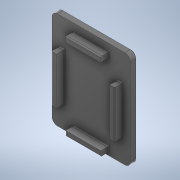
# Autodesk Inventor part: SP19V1 Tapacanto Delantero
Saved by Autodesk Inventor 2021.2 (Build 252289000, 289)
## iProperties
Created: 2026-06-08
Part Number: SP19V1 Tapacanto Delantero
Material: ABS Plastic
Document SubType Name: Modeling
Designer: NELSON
Density: 1.06 g/cm^3
Appearance: Smooth - Black
Author: NELSON
Autodesk Inventor part; units mm, degrees
ref_plane "YZ Plane" through (0, 0, 0) normal (1, 0, 0) x (0, 1, 0)
ref_plane "XZ Plane" through (0, 0, 0) normal (0, 1, 0) x (-1, 0, 0)
ref_plane "XY Plane" through (0, 0, 0) normal (0, 0, 1) x (1, 0, 0)
sketch "Boceto1" plane through (0, 0, 0) normal (0, 0, 1) x (1, 0, 0)
  line L0 (30, -40) -> (-30, -40)
  line L1 (-30, -40) -> (-30, 40)
  line L2 (-30, 40) -> (30, 40)
  line L3 (30, 40) -> (30, -40)
  line L4 (30, -40) -> (-30, 40) construction
  line L5 (-30, -40) -> (30, 40) construction
  line L6 (33.7, -43.7) -> (-33.7, -43.7)
  line L7 (-33.7, -43.7) -> (-33.7, 43.7)
  line L8 (-33.7, 43.7) -> (33.7, 43.7)
  line L9 (33.7, 43.7) -> (33.7, -43.7)
  line L10 (-33.7, -40) -> (33.7, -40)
  point P0 (0, 0)
  point P1 (30, -40)
  point P2 (-30, -40)
  dimension "d0" = 60
  dimension "d1" = 80
  dimension "d2" = 3.7
  dimension "d20" = 3.7
  constraints: 22 end point, 4 parallel, 3 perpendicular, 2 midpoint, 2 point on line, 1 horizontal, 3 other
  measures "d0" distance of L1.end L2.end
  measures "d1" distance of L0.end L1.end
  measures "d2" distance between parallel lines of L3 L9
  measures "d20" distance between parallel lines of L6 L10
extrude "Extrusión1" add sketch "Boceto1" along normal blind 5 contours L0 L1 L2 L3 | L3 L2 L1 L10 L7 L8 L9
sketch "Boceto2" plane through (0, 0, 5) normal (0, 0, 1) x (1, 0, 0)
  line L0 (-27.48, -37.48) -> (27.48, -37.48)
  line L1 (27.48, -37.48) -> (27.48, 37.48)
  line L2 (27.48, 37.48) -> (-27.48, 37.48)
  line L3 (-27.48, 37.48) -> (-27.48, -37.48)
  line L4 (-27.48, -37.48) -> (27.48, 37.48) construction
  line L5 (27.48, -37.48) -> (-27.48, 37.48) construction
  line L6 (-27.08, 37.08) -> (27.08, 37.08)
  line L7 (27.08, 37.08) -> (27.08, -37.08)
  line L8 (27.08, -37.08) -> (-27.08, -37.08)
  line L9 (-27.08, -37.08) -> (-27.08, 37.08)
  line L10 (-27.08, 0) -> (-25.08, 0)
  line L11 (-23.08, -20) -> (-27.08, -20)
  line L12 (-27.08, -20) -> (-27.08, 20)
  line L13 (-27.08, 20) -> (-23.08, 20)
  line L14 (-23.08, 20) -> (-23.08, -20)
  line L15 (-23.08, -20) -> (-27.08, 20) construction
  line L16 (-27.08, -20) -> (-23.08, 20) construction
  line L17 (0, 0) -> (0, 2.2865)
  line L18 (0, 0) -> (-1.3296, 0)
  line L19 (23.08, -20) -> (27.08, -20)
  line L20 (27.08, -20) -> (27.08, 20)
  line L21 (27.08, 20) -> (23.08, 20)
  line L22 (23.08, 20) -> (23.08, -20)
  line L23 (23.08, -20) -> (27.08, 20) construction
  line L24 (27.08, -20) -> (23.08, 20) construction
  line L25 (0, 37.08) -> (0, 35.08)
  line L26 (15, 33.08) -> (-15, 33.08)
  line L27 (-15, 33.08) -> (-15, 37.08)
  line L28 (-15, 37.08) -> (15, 37.08)
  line L29 (15, 37.08) -> (15, 33.08)
  line L30 (15, 33.08) -> (-15, 37.08) construction
  line L31 (-15, 33.08) -> (15, 37.08) construction
  line L32 (15, -33.08) -> (-15, -33.08)
  line L33 (-15, -33.08) -> (-15, -37.08)
  line L34 (-15, -37.08) -> (15, -37.08)
  line L35 (15, -37.08) -> (15, -33.08)
  line L36 (15, -33.08) -> (-15, -37.08) construction
  line L37 (-15, -33.08) -> (15, -37.08) construction
  point P0 (25.08, 0)
  point P1 (0, -35.08)
  dimension "d25" = 54.96
  dimension "d26" = 74.96
  dimension "d27" = 0.4
  dimension "d28" = 2
  dimension "d29" = 40
  dimension "d30" = 2
  dimension "d31" = 30
  constraints: 76 end point, 12 midpoint, 10 symmetric about line, 8 parallel, 5 horizontal, 4 perpendicular, 2 point on line, 2 vertical, 3 other
  measures "d25" distance of L2.end L1.end
  measures "d26" distance of L1.end L0.end
  measures "d27" distance between parallel lines of L2 L6
  measures "d28" distance of L10.start L10.end
  measures "d29" distance of L11.end L12.end
  measures "d30" distance of L25.start L25.end
  measures "d31" distance of L27.end L28.end
extrude "Extrusión2" add sketch "Boceto2" along normal blind 7 draft 2 contours L6 L29 L26 L27 | L13 L14 L11 L9 | L7 L19 L22 L21 | L33 L32 L35 L8
fillet "Empalme1" radius 4.716 4 edges at (33.7, 43.7, 2.5) (-33.7, 43.7, 2.5) (33.7, -40, 2.5) (-33.7, -40, 2.5)
fillet "Empalme1" radius 1 15 edges at (0, 37.3244, 12) (27.3244, 0, 12) (0, -37.3244, 12) (-27.3244, 0, 12) (-23.08, 0, 5) (0, 33.08, 5) (0, -33.08, 5) (15, -35.08, 5) (-25.08, -20, 5) (-25.08, 20, 5) (-15, 35.08, 5) (15, 35.08, 5) (25.08, 20, 5) (25.08, -20, 5) (-15.2444, -35.08, 12)
chamfer "Chamfer1" distance 0.3 angle 45 8 edges at (0, 43.7, 0) (-32.3187, 42.3187, 0) (-33.7, 1.85, 0) (-32.3187, -38.6187, 0) (0, -40, 0) (32.3187, -38.6187, 0) (33.7, 1.85, 0) (32.3187, 42.3187, 0)
